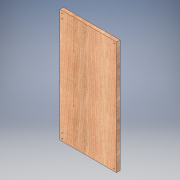
# Autodesk Inventor part: Middle Board
Saved by Autodesk Inventor 2018 (Build 220112000, 112)
## iProperties
Created: 2018-12-30
Part Number: Middle Board
Material: Generic
Document SubType Name: Modeling
Designer: maste
Density: 1 g/cm^3
Appearance: Default
Author: maste
Autodesk Inventor part; units mm, degrees
ref_plane "YZ Plane" through (0, 0, 0) normal (1, 0, 0) x (0, 1, 0)
ref_plane "XZ Plane" through (0, 0, 0) normal (0, 1, 0) x (-1, 0, 0)
ref_plane "XY Plane" through (0, 0, 0) normal (0, 0, 1) x (1, 0, 0)
sketch "Sketch1" plane through (0, 0, 0) normal (0, 0, 1) x (1, 0, 0)
  line L0 (0, 0) -> (304.8, 0)
  line L1 (304.8, 0) -> (304.8, 609.6)
  line L2 (304.8, 609.6) -> (0, 609.6)
  line L3 (0, 609.6) -> (0, 0)
  dimension "d0" = 304.8
  dimension "d1" = 609.6
  constraints: 8 end point, 2 parallel, 1 horizontal, 1 perpendicular
  measures "d0" distance of L2.end L1.end
  measures "d1" distance of L1.end L0.end
extrude "Extrusion1" add sketch "Sketch1" along normal blind 19.05
sketch "Sketch2" plane through (0, 0, 19.05) normal (0, 0, 1) x (1, 0, 0)
  line L0 (0, 0) -> (12.7, 0) construction
  line L1 (12.7, 0) -> (0, 0) construction
  line L2 (0, 0) -> (304.8, 0) construction
  line L3 (12.7, 0) -> (0, 0) construction
  line L4 (0, 0) -> (0, 12.7) construction
  line L5 (0, 609.6) -> (0, 0) construction
  line L6 (0, 12.7) -> (12.7, 12.7) construction
  circle A0 centre (12.7, 12.7) radius 2.5797
  line L7 (304.8, 0) -> (304.8, 609.6) construction
  line L8 (304.8, 304.8) -> (0, 304.8) construction
  line L9 (152.4, 0) -> (152.4, 609.6) construction
  line L10 (304.8, 609.6) -> (0, 609.6) construction
  circle A1 centre (12.7, 596.9) radius 2.5797
  circle A2 centre (292.1, 12.7) radius 2.5797
  circle A3 centre (292.1, 596.9) radius 2.5797
  line L11 (12.7, 596.9) -> (12.7, 571.5) construction
  circle A4 centre (12.7, 571.5) radius 2.5797
  circle A5 centre (12.7, 38.1) radius 2.5797
  dimension "d4" = 12.7
  dimension "d5" = 12.7
  dimension "d6" = 12.7
  dimension "d7" = 12.7
  dimension "d8" = 5.1594
  dimension "d11" = 25.4
  constraints: 16 end point, 6 centre point, 4 midpoint, 4 symmetric about line, 2 coincident, 1 collinear, 1 perpendicular, 1 point on line, 1 vertical, 4 other
  measures "d4" distance of L0.start L0.end
  measures "d5" distance of L0.end L0.start
  measures "d6" distance of L0.end L0.start
  measures "d7" distance of L0.start L4.end
  measures "d8" diameter of A0
  measures "d11" distance of L11.start L11.end
extrude "Extrusion3" cut sketch "Sketch2" against normal blind 19.05
body "Solid1"
